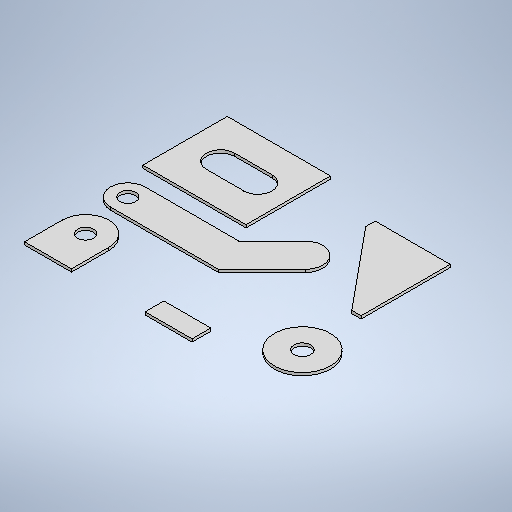
# Autodesk Inventor part: rings
Saved by Autodesk Inventor 2025.3 (Build 293356030, 356C)
## iProperties
Created: 2025-09-01
Part Number: rings
Material: Stainless Steel
Document SubType Name: Sheet Metal
Designer: admin
Mass: 280.619 g
Surface Area: 364.406 cm^2
Volume: 35.0774 cm^3
Density: 8 g/cm^3
Sheet Metal Rule: AISI304 3mm Die 32
Sheet Metal Width: 90,000 mm
Sheet Metal Length: 110,000 mm
Sheet Metal Area: 9900,000 mm^2
Appearance: Default
Flat Pattern Width: 9 cm
Flat Pattern Length: 11 cm
Flat Pattern Area: 99 cm^2
Author: admin
Autodesk Inventor part; units mm, degrees
ref_plane "YZ Plane" through (0, 0, 0) normal (1, 0, 0) x (0, 1, 0)
ref_plane "XZ Plane" through (0, 0, 0) normal (0, 1, 0) x (-1, 0, 0)
ref_plane "XY Plane" through (0, 0, 0) normal (0, 0, 1) x (1, 0, 0)
sketch "Sketch1" plane through (0, 0, 0) normal (0, 0, 1) x (1, 0, 0)
  line L0 (0, 0) -> (50, 0)
  line L1 (50, 0) -> (50, 20)
  line L2 (50, 20) -> (0, 20)
  line L3 (0, 20) -> (0, 0)
  line L4 (-15.3259, 115.323) -> (-115.3259, 115.323)
  arc A0 (-115.3259, 115.323) -> (-115.3259, 78.323) centre (-115.3259, 96.823) ccw
  line L5 (-115.3259, 78.323) -> (0, 78.323)
  line L6 (0, 78.323) -> (46.1924, 124.5154)
  arc A1 (46.1924, 124.5154) -> (20.0294, 150.6784) centre (33.1109, 137.5969) ccw
  line L7 (20.0294, 150.6784) -> (-15.3259, 115.323)
  circle A2 centre (-115.3259, 96.823) radius 8.5
  line L8 (0, 0) -> (0, 78.323) construction
  circle A3 centre (-103.9405, 40.3629) radius 8.5
  line L9 (-128.9405, 0.3629) -> (-128.9405, 40.3629)
  arc A4 (-78.9405, 40.3629) -> (-128.9405, 40.3629) centre (-103.9405, 40.3629) ccw
  line L10 (-78.9405, 40.3629) -> (-78.9405, 0.3629)
  line L11 (-78.9405, 0.3629) -> (-128.9405, 0.3629)
  line L12 (38.8442, 206.4801) -> (118.8442, 206.4801)
  line L13 (118.8442, 206.4801) -> (118.8442, 111.4801)
  line L14 (38.8442, 206.4801) -> (38.8442, 196.4801)
  line L15 (118.8442, 111.4801) -> (108.8442, 111.4801)
  line L16 (108.8442, 111.4801) -> (38.8442, 196.4801)
  line L17 (-136.6803, 224.2575) -> (-26.6803, 224.2575)
  line L18 (-26.6803, 224.2575) -> (-26.6803, 134.2575)
  line L19 (-26.6803, 134.2575) -> (-136.6803, 134.2575)
  line L20 (-136.6803, 134.2575) -> (-136.6803, 224.2575)
  line L21 (-98.9405, 179.2575) -> (-58.9405, 179.2575) construction
  line L22 (-98.9405, 194.2575) -> (-58.9405, 194.2575)
  line L23 (-58.9405, 164.2575) -> (-98.9405, 164.2575)
  arc A5 (-98.9405, 194.2575) -> (-98.9405, 164.2575) centre (-98.9405, 179.2575) ccw
  arc A6 (-58.9405, 164.2575) -> (-58.9405, 194.2575) centre (-58.9405, 179.2575) ccw
  circle A7 centre (118.8442, 48.8629) radius 30
  circle A8 centre (118.8442, 48.8629) radius 9
  line L24 (-136.6803, 218.2575) -> (-26.6803, 218.2575) construction
  point P0 (-78.9405, 179.2575)
  dimension "d22" = 50
  dimension "d23" = 20
  dimension "d24" = 17
  dimension "d25" = 10
  dimension "d26" = 100
  dimension "d28" = 135
  dimension "d29" = 50
  dimension "d30" = 17
  dimension "d31" = 25
  dimension "d32" = 40
  dimension "d33" = 80
  dimension "d34" = 95
  dimension "d35" = 10
  dimension "d36" = 10
  dimension "d37" = 110
  dimension "d38" = 30
  dimension "d39" = 40
  dimension "d40" = 60
  dimension "d41" = 18
  dimension "d42" = 6
  dimension "d43" = 90
  measures "d22" distance of L2.end L1.end
  measures "d23" distance of L1.end L0.end
  measures "d24" diameter of A2
  measures "d25" radial gap between concentric circles of A0 A2
  measures "d26" horizontal distance of A0.centre L4.start
  measures "d28" angle of L4 L7
  measures "d29" distance of L7.start L4.start
  measures "d30" diameter of A3
  measures "d31" radius of A4
  measures "d32" distance of L10.start L10.end
  measures "d33" distance of L12.start L12.end
  measures "d34" distance of L12.end L13.end
  measures "d35" distance of L12.start L14.end
  measures "d36" distance of L13.end L15.end
  measures "d37" distance of L17.start L17.end
  measures "d38" distance between parallel lines of L23 L22
  measures "d39" distance of L21.start L21.end
  measures "d40" diameter of A7
  measures "d41" diameter of A8
  measures "d42" distance between parallel lines of L24 L17
  measures "d43" distance of L19.end L17.start
extrude "Plate1" add sketch "Sketch1" along normal blind 3
equation "\"d2\" = Thickness"
equation "\"BendReliefWidth\" = Thickness"
equation "\"BendReliefDepth\" = 0.5 * Thickness"
equation "\"CornerReliefSize\" = 4 * Thickness"
equation "\"MinimumRemnant\" = 2 * Thickness"
equation "\"TransitionRadius\" = BendRadius"
equation "\"JacobiRadiusSize\" = BendRadius"
equation "\"GapSize\" = Thickness"
equation "\"Thickness\" = 3"
equation "\"BendRadius\" = 5"
body "Solid1"
